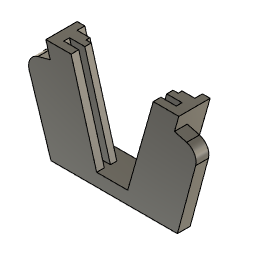
Power steering reservoir holder v1 (Autodesk Fusion 360 design; units mm, degrees)
Autodesk Fusion 360 part; units mm, degrees
note: some values were not read from the file. Set by a fixed rule: which sketch regions a step uses.
sketch "Sketch1" plane through (0, 0, 0) normal (0, 0, 1) x (1, 0, 0)
  line L0 (0, 12.25) -> (0, 0)
  line L1 (22, 5.25) -> (22, 7.75)
  line L2 (26, 5.25) -> (22, 5.25)
  line L3 (22, 7.75) -> (24, 7.75)
  line L4 (10, 5.25) -> (10, 7.75)
  line L5 (10, 7.75) -> (8, 7.75)
  line L6 (8, 7.75) -> (8, 9.25)
  line L7 (6, 3) -> (26, 3)
  line L8 (6, 5.25) -> (10, 5.25)
  line L9 (5, 12.25) -> (0, 12.25)
  line L10 (32, 12.25) -> (32, 0)
  line L11 (24, 9.25) -> (27, 9.25)
  line L12 (8, 9.25) -> (5, 9.25)
  line L13 (0, 0) -> (32, 0)
  line L14 (16, 3) -> (16, 20.1326) construction
  line L15 (24, 7.75) -> (24, 9.25)
  line L16 (27, 12.25) -> (32, 12.25)
  line L17 (9.867, 3) -> (9.867, 0)
  line L18 (5, 12.25) -> (27, 12.25)
  line L19 (22, 3) -> (22, 0)
  line L20 (26, 5.25) -> (28, 5.25)
  line L21 (28, 5.25) -> (28, 3)
  line L22 (28, 3) -> (26, 3)
  line L23 (4, 5.25) -> (4, 3)
  line L24 (6, 5.25) -> (4, 5.25)
  line L25 (4, 3) -> (6, 3)
  line L26 (27, 9.25) -> (29, 9.25)
  line L27 (29, 9.25) -> (29, 12.25)
  line L28 (3, 9.25) -> (3, 12.25)
  line L29 (5, 9.25) -> (3, 9.25)
  dimension "d12" = 4
  dimension "d13" = 2.5
  dimension "d14" = 2
  dimension "d15" = 1.5
  dimension "d16" = 3
  dimension "d17" = 3
  dimension "d40" = 2
  dimension "d42" = 2.25
  constraint horizontal L7
  constraint perpendicular L1 L2
  constraint perpendicular L1 L3
  constraint perpendicular L3 L15
  constraint perpendicular L11 L15
  constraint midpoint L14.start L7
  constraint perpendicular L7 L14
  constraint perpendicular L10 L16
  constraint symmetric L2.start L8.start L14
  constraint symmetric L1.start L4.start L14
  constraint symmetric L1.end L4.end L14
  constraint symmetric L5.end L3.end L14
  constraint symmetric L11.start L6.end L14
  constraint symmetric L11.end L12.end L14
  constraint symmetric L16.start L9.start L14
  constraint symmetric L0.start L10.start L14
  constraint symmetric L0.end L10.end L14
  constraint coincident L7 L17.start
  constraint coincident L13 L17.end
  constraint perpendicular L13 L17
  constraint coincident L0.end L13.start
  constraint coincident L7 L19.start
  constraint coincident L13 L19.end
  constraint perpendicular L13 L19
  constraint parallel L2 L20
  constraint perpendicular L7 L21
  constraint perpendicular L21 L22
  constraint symmetric L2.start L14 L8.start
  constraint symmetric L7.end L14 L7.start
  constraint symmetric L14 L20.end L23.start
  constraint symmetric L14 L21.end L23.end
  constraint horizontal L26
  constraint coincident L16 L27.end
  constraint perpendicular L16 L27
  constraint symmetric L11.end L14 L12.end
  constraint symmetric L14 L26.end L28.start
  constraint symmetric L14 L27.end L28.end
  measures "d12" distance of L1.start L2.start
  measures "d13" distance of L1.end L1.start
  measures "d14" distance of L1.end L3.end
  measures "d15" distance of L11.start L3.end
  measures "d16" distance of L11.start L11.end
  measures "d17" distance of L11.end L16.start
  measures "d40" distance of L11.end L26.end
  measures "d42" distance of L20.end L21.end
sketch "Sketch4" plane through (0, 0, 0) normal (0, 1, 0) x (1, 0, 0)
  line L0 (6, 0) -> (26, 0)
  line L1 (6, 0) -> (6, -35) construction
  line L2 (16, -35.0084) -> (-3.5, -35.0084) construction
  line L3 (16, 0) -> (16, -35.0084) construction
  line L4 (26, 0) -> (26, -35) construction
  line L5 (16, 0) -> (26, -35)
  line L6 (16, 0) -> (6, -35)
  constraint coincident L0.start L1.start
  constraint perpendicular L0 L1
  constraint perpendicular L1 L2
  constraint midpoint L0 L3.start
  constraint perpendicular L2 L3
  constraint symmetric L0.start L3 L0.end
  constraint symmetric L1.end L3 L4.end
  constraint symmetric L5.start L3 L6.start
  constraint symmetric L3 L4.end L1.end
sweep "Sweep1" add profiles "Sketch1" path "Sketch4" along L6 section 1 contours L0 L4 L5 L6 L7 L8 L9 L12 L13 L17 L23 L24 L25 L28 L29
extrude "Extrude1" add sketch "Sketch1" against normal blind 5
sweep "Sweep2" add profiles "Sketch1" path "Sketch4" along L5 section 1 contours L1 L2 L3 L7 L10 L11 L13 L15 L16 L19 L20 L21 L22 L26 L27
sketch "Sketch5" plane through (0, 0, 0) normal (0, -1, 0) x (1, 0, 0)
  line L0 (-0.133, 35) -> (-10, 35)
  line L1 (0, 0) -> (0, -5)
  line L2 (0, -5) -> (32, -5)
  line L3 (32, -5) -> (32, 0)
  line L4 (32, 0) -> (42, 35)
  line L5 (42, 35) -> (32, 35)
  line L6 (32, 35) -> (22, 0)
  line L7 (22, 0) -> (9.867, 0)
  circle A0 centre (-11.7548, 22.9097) radius 5
  line L8 (-13.0636, 27.7353) -> (-8.294, 29.029)
  line L9 (-5.5936, 19.5776) -> (-10.2811, 18.1318)
  line L10 (16, 0) -> (16, 35.0084)
  line L11 (9.867, 0) -> (-0.133, 35)
  line L12 (-10, 35) -> (0, 0)
  line L13 (37.5936, 19.5776) -> (42.2811, 18.1318)
  circle A1 centre (43.7548, 22.9097) radius 5
  line L14 (45.0636, 27.7353) -> (40.294, 29.029)
  line L15 (16, -5) -> (20.8519, -5)
  line L16 (0, -5) -> (-7.9856, -5)
  line L17 (32, -5) -> (41.4479, -5)
  line L18 (48.5842, 21.6147) -> (41.4479, -5)
  line L19 (-16.5123, 21.3714) -> (-7.9856, -5)
  dimension "d43" = 10
  constraint coincident A0 L8.start
  constraint tangent A0 L8
  constraint coincident A0 L9.end
  constraint tangent A0 L9
  constraint coincident L12 L8.end
  constraint coincident L12 L9.start
  constraint symmetric A0 L10 A1
  constraint symmetric L8.start L10 L14.start
  constraint symmetric L9.end L10 L13.end
  constraint symmetric L10 L8.end L14.end
  constraint symmetric L10 L9.start L13.start
  constraint midpoint L2 L15.start
  constraint coincident L2 L15.end
  constraint coincident L1.end L2.start
  constraint perpendicular L1 L16
  constraint coincident L2.end L3.start
  constraint perpendicular L3 L17
  constraint coincident A1 L18.start
  constraint coincident L17 L18.end
  constraint tangent A1 L18
  constraint coincident A0 L19.start
  constraint coincident L16 L19.end
  constraint tangent A0 L19
  measures "d43" diameter of A0
extrude "Extrude2" add sketch "Sketch5" against normal blind 5 contours A0 L8 L9 L12 | A0 | L1 A0 L9 L12 L16 L19 | L4 L13 A1 L14 | L3 L4 L13 A1 L17 L18 | A1
